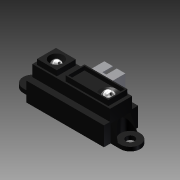
# Autodesk Inventor part: SharpIRsensor
Saved by Autodesk Inventor 2016 (Build 200138000, 138)
## iProperties
Created: 2012-10-14
Part Number: SharpIRsensor
Material: Ogólny
Document SubType Name: Modeling
Designer: ZSSD
Density: 1 g/cm^3
Appearance: Domyślna
Author: ZSSD
Autodesk Inventor part; units mm, degrees
sketch "Sketch1" plane through (0, 0, 0) normal (0, 0, 1) x (1, 0, 0)
  line L0 (0, 0) -> (29.5, 0)
  line L1 (29.5, 0) -> (29.5, 13)
  line L2 (29.5, 13) -> (0, 13)
  line L3 (0, 13) -> (0, 0)
  dimension "d0" = 29.5
  dimension "d1" = 13
  constraints: 8 end point, 2 parallel, 1 horizontal, 1 perpendicular
  measures "d0" distance of L2.end L1.end
  measures "d1" distance of L0.end L1.end
extrude "Extrusion1" add sketch "Sketch1" along normal blind 13.5
sketch "Sketch2" plane through (0, 0, 13.5) normal (0, 0, 1) x (1, 0, 0)
  line L0 (0, 0) -> (0, 13) projected
  line L1 (29.5, 13) -> (29.5, 0) projected
  line L2 (0, 6.5) -> (29.5, 6.5)
  line L3 (29.5, 6.5) -> (29.5, 10.7)
  line L4 (29.5, 10.7) -> (0, 10.7)
  line L5 (0, 10.7) -> (0, 6.5)
  line L6 (29.5, 10.7) -> (0, 10.7)
  line L7 (0, 10.7) -> (0, 2.3)
  line L8 (0, 2.3) -> (29.5, 2.3)
  line L9 (29.5, 2.3) -> (29.5, 10.7)
  dimension "d4" = 4.2
  dimension "d5" = 8.4
  constraints: 16 end point, 4 parallel, 2 horizontal, 2 perpendicular, 2 point on line, 1 midpoint
  measures "d4" distance of L3.end L2.end
  measures "d5" distance of L7.end L6.end
extrude "Extrusion2" add sketch "Sketch2" along normal blind 6.3
sketch "Sketch3" plane through (0, 0, 19.8) normal (0, 0, 1) x (1, 0, 0)
  line L0 (0, 2.3) -> (0, 10.7) projected
  line L1 (29.5, 2.3) -> (0, 2.3) projected
  line L2 (29.5, 10.7) -> (29.5, 2.3) projected
  line L3 (0, 10.7) -> (29.5, 10.7) projected
  line L4 (29.5, 6.5) -> (0, 6.5)
  line L5 (0, 6.5) -> (0, 10.1)
  line L6 (0, 10.1) -> (29.5, 10.1)
  line L7 (29.5, 10.1) -> (29.5, 6.5)
  line L8 (0, 10.1) -> (29.5, 10.1)
  line L9 (29.5, 10.1) -> (29.5, 2.9)
  line L10 (29.5, 2.9) -> (0, 2.9)
  line L11 (0, 2.9) -> (0, 10.1)
  line L12 (0, 10.7) -> (29.5, 10.7)
  line L13 (29.5, 10.7) -> (29.5, 10.1)
  line L14 (29.5, 10.1) -> (0, 10.1)
  line L15 (0, 10.1) -> (0, 10.7)
  point P0 (0, 0)
  dimension "d8" = 3.6
  dimension "d9" = 7.2
  constraints: 24 end point, 6 parallel, 3 horizontal, 3 perpendicular, 2 point on line, 1 midpoint
  measures "d8" distance of L4.end L5.end
  measures "d9" distance of L8.end L9.end
extrude "Extrusion3" cut sketch "Sketch3" against normal blind 2 contours L0 L10 L2 L1 | L0 L3 L2 L6
sketch "Sketch4" plane through (0, 0, 19.8) normal (0, 0, 1) x (1, 0, 0)
  line L0 (29.5, 10.1) -> (0, 10.1) projected
  line L1 (0, 2.9) -> (29.5, 2.9) projected
  line L2 (29.5, 2.9) -> (28.3, 2.9)
  line L3 (28.3, 2.9) -> (28.3, 10.1)
  line L4 (28.3, 10.1) -> (29.5, 10.1)
  line L5 (29.5, 10.1) -> (29.5, 2.9)
  line L6 (0, 10.1) -> (1.2, 10.1)
  line L7 (1.2, 10.1) -> (1.2, 2.9)
  line L8 (1.2, 2.9) -> (0, 2.9)
  line L9 (0, 2.9) -> (0, 10.1)
  point P0 (0, 0)
  dimension "d12" = 1.2
  dimension "d13" = 1.2
  constraints: 16 end point, 4 parallel, 2 horizontal, 2 perpendicular, 2 point on line
  measures "d12" distance of L3.end L4.end
  measures "d13" distance of L7.end L8.end
extrude "Extrusion4" cut sketch "Sketch4" against normal blind 2 contours L5 L1 L3 L0 | L7 L1 L9 L0
sketch "Sketch5" plane through (0, 0, 19.8) normal (0, 0, 1) x (1, 0, 0)
  line L0 (1.2, 2.9) -> (28.3, 2.9) projected
  line L1 (28.3, 10.1) -> (12, 10.1)
  line L2 (12, 10.1) -> (12, 2.9)
  line L3 (12, 2.9) -> (28.3, 2.9)
  line L4 (28.3, 2.9) -> (28.3, 10.1)
  line L5 (1.2, 10.1) -> (8.7, 10.1)
  line L6 (8.7, 10.1) -> (8.7, 2.9)
  line L7 (8.7, 2.9) -> (1.2, 2.9)
  line L8 (1.2, 2.9) -> (1.2, 10.1)
  line L9 (8.7, 10.1) -> (12, 10.1)
  line L10 (12, 10.1) -> (12, 2.9)
  line L11 (12, 2.9) -> (8.7, 2.9)
  line L12 (8.7, 2.9) -> (8.7, 10.1)
  point P0 (0, 0)
  dimension "d16" = 16.3
  dimension "d17" = 7.5
  constraints: 24 end point, 6 parallel, 3 horizontal, 3 perpendicular, 2 point on line
  measures "d16" distance of L3.end L2.end
  measures "d17" distance of L6.end L7.end
extrude "Extrusion5" cut sketch "Sketch5" against normal up to surface (2 mm away) contours L6 L9 L2 L0
sketch "Sketch6" plane through (0, 0, 0) normal (0, 0, -1) x (-1, 0, 0)
  line L0 (0, 0) -> (-29.5, 0) projected
  line L1 (0, 13) -> (0, 0) projected
  line L2 (-29.5, 13) -> (0, 13) projected
  line L3 (-29.5, 0) -> (-29.5, 13) projected
extrude "Extrusion6" cut sketch "Sketch6" against normal blind 6.3
sketch "Sketch7" plane through (0, 0, 6.3) normal (0, 0, -1) x (-1, 0, 0)
  line L0 (-29.5, 0) -> (-29.5, 13) projected
  line L1 (0, 0) -> (-29.5, 0) projected
  line L2 (-29.5, 6.2731) -> (-33.25, 6.2731)
  circle A0 centre (-33.25, 6.2731) radius 3.75
  circle A1 centre (-33.25, 6.2731) radius 1.6
  line L3 (-33.25, 10.0231) -> (-29.5, 10.0231)
  line L4 (-33.25, 2.5231) -> (-29.5, 2.5231)
  dimension "d22" = 3.75
  dimension "d23" = 3.2
  constraints: 6 end point, 3 point on circle, 3 point on line, 2 centre point, 2 coincident, 2 perpendicular, 2 tangent, 1 parallel
  measures "d22" distance of L2.start L2.end
  measures "d23" diameter of A1
extrude "Extrusion7" add sketch "Sketch7" against normal blind 1.5
sketch "Sketch8" plane through (0, 0, 7.8) normal (0, 0, 1) x (1, 0, 0)
  circle A0 centre (33.25, 6.2731) radius 1.6 projected
  line L0 (29.5, 10.0231) -> (33.25, 10.0231) projected
  line L1 (29.5, 2.5231) -> (29.5, 10.0231) projected
  line L2 (33.25, 2.5231) -> (29.5, 2.5231) projected
  arc A1 (33.25, 2.5231) -> (33.25, 10.0231) centre (33.25, 6.2731) ccw projected
  line L3 (29.5, 6.2731) -> (37, 6.2731)
  line L4 (33.25, 6.2731) -> (29.5, 6.2731)
  line L5 (29.5, 6.2731) -> (32.1, 6.2731)
  line L6 (32.1, 2.5231) -> (32.1, 10.0231)
  point P0 (0, 0)
  dimension "d26" = 2.6
  constraints: 8 end point, 3 point on line, 1 collinear, 1 midpoint, 1 perpendicular, 1 point on circle
  measures "d26" distance of L3.start L5.end
sketch "Sketch9" plane through (29.5, 10.7, 13.5) normal (1, 0, 0) x (0, 0, -1)
  line L0 (7.2, -8.1769) -> (5.7, -8.1769) projected
  line L1 (5.7, -8.1769) -> (5.7, -0.6769) projected
  line L2 (5.7, -0.6769) -> (7.2, -0.6769) projected
  line L3 (7.2, -0.6769) -> (7.2, 2.3) projected
  line L4 (7.2, 2.3) -> (0, 2.3) projected
  line L5 (0, 2.3) -> (0, 0) projected
  line L6 (0, 0) -> (-4.3, 0) projected
  line L7 (-4.3, 0) -> (-4.3, -8.4) projected
  line L8 (0, -8.4) -> (-4.3, -8.4) projected
  line L9 (0, -8.4) -> (0, -10.7) projected
  line L10 (7.2, -10.7) -> (0, -10.7) projected
  line L11 (7.2, -10.7) -> (7.2, -8.1769) projected
  line L12 (5.7, -8.1769) -> (0.7, -8.1769)
  line L13 (0.7, -8.1769) -> (0.7, -1.0276)
  line L14 (0.7, -1.0276) -> (5.7, -1.0276)
  line L15 (5.7, -1.0276) -> (5.7, -8.1769)
  point P0 (13.5, -10.7)
  dimension "d27" = 5
  constraints: 8 end point, 2 parallel, 1 horizontal, 1 perpendicular
  measures "d27" distance of L13.end L14.end
ref_plane "Work Plane1" through (31.375, 2.5231, 7.8) normal (0, -1, 0) x (1, 0, 0)
sketch "Sketch10" plane through (31.375, 2.5231, 7.8) normal (0, -1, 0) x (1, 0, 0)
  line L0 (-1.875, 0) -> (-1.875, 5) projected
  line L1 (1.875, 0) -> (-1.875, 0) projected
  line L2 (-1.875, 5) -> (0.725, 0)
  point P0 (-31.375, -7.8)
  constraints: 2 end point
extrude "Extrusion8" add sketch "Sketch10" against normal up to surface (7.5 mm away)
sketch "Sketch11" plane through (0, 0, 7.8) normal (0, 0, 1) x (1, 0, 0)
  arc A0 (33.25, 2.5231) -> (33.25, 10.0231) centre (33.25, 6.2731) ccw projected
  circle A1 centre (33.25, 6.2731) radius 3.75
  point P0 (0, 0)
  constraints: 1 centre point, 1 coincident, 1 concentric
extrude "Extrusion9" cut sketch "Sketch11" along normal through all
ref_plane "Work Plane2" through (14.75, 0, 13.5) normal (1, 0, 0) x (0, 0, -1)
mirror "Mirror1" about plane through (14.75, 0, 13.5) normal (1, 0, 0) of "Extrusion9", "Extrusion8", "Extrusion7"
sketch "Sketch12" plane through (0, 0, 19.8) normal (0, 0, 1) x (1, 0, 0)
  line L0 (1.2, 2.9) -> (8.7, 2.9) projected
  line L1 (4.95, 2.9) -> (4.95, 3.9)
  circle A0 centre (4.95, 6.5) radius 2.6
  point P0 (0, 0)
  dimension "d32" = 1
  constraints: 2 end point, 1 midpoint, 1 perpendicular, 1 vertical alignment, 2 other
  measures "d32" distance of L1.start L1.end
sketch "Sketch13" plane through (0, 0, 17.8) normal (0, 0, 1) x (1, 0, 0)
  circle A0 centre (4.95, 6.5) radius 1.75
  point P0 (0, 0)
  dimension "d33" = 3.5
  constraints: 1 centre point
  measures "d33" diameter of A0
loft "Loft1" cut profiles "Sketch13", "Sketch12"
sketch "Sketch14" plane through (4.95, 6.5, 17.8) normal (0, 0, 1) x (1, 0, 0)
  circle A0 centre (0, 0) radius 1.75 projected
  line L0 (-1.75, 0) -> (1.75, 0)
  point P0 (-4.95, -6.5)
  constraints: 2 end point, 2 point on circle, 1 horizontal
ref_plane "Work Plane3" through (0, 6.5, 13.5) normal (0, -1, 0) x (1, 0, 0)
sketch "Sketch15" plane through (0, 6.5, 13.5) normal (0, -1, 0) x (1, 0, 0)
  line L0 (3.2, 4.3) -> (6.7, 4.3) projected
  line L1 (3.2, 4.3) -> (6.7, 4.3)
  circle A0 centre (4.95, 4.3) radius 1.7743
  line L2 (6.7, 4.3) -> (3.1757, 4.3)
  arc A1 (6.7, 4.3) -> (3.1757, 4.3) centre (4.9379, 4.3121) ccw
  point P0 (0, -13.5)
  constraints: 4 end point, 2 point on circle, 1 centre point, 1 collinear, 1 horizontal alignment, 1 midpoint, 2 other
revolve "Revolution1" add sketch "Sketch15" angle 90 about axis through (3.2, 6.5, 17.8) along (1, 0, 0) picked at (5.5194, 4.4315) contours L2 A0 A1 L0 | A1 A0
sketch "Sketch16" plane through (3.2, 6.5, 17.8) normal (0, 1, 0) x (1, 0, 0)
  line L0 (-0.0238, -0.0559) -> (0, 0) projected
  arc A0 (-0.0238, -0.0559) -> (3.5, 0) centre (1.7379, -0.0121) ccw projected
  line L1 (0, 0) -> (3.5, 0) projected
  point P0 (-3.2, 17.8)
revolve "Revolution2" add sketch "Sketch16" angle 90 about axis through (3.2, 6.5, 17.8) along (-1, 0, 0)
sketch "Sketch17" plane through (0, 0, 19.8) normal (0, 0, 1) x (1, 0, 0)
  line L0 (12, 10.1) -> (12, 2.9) projected
  line L1 (12, 2.9) -> (28.3, 2.9) projected
  line L2 (28.3, 2.9) -> (28.3, 10.1) projected
  line L3 (28.3, 10.1) -> (12, 10.1) projected
  line L4 (13.3298, 10.1) -> (13.3298, 9.6)
  line L5 (12, 6.5) -> (12.5, 6.5)
  line L6 (25.802, 2.9) -> (25.802, 3.4)
  line L7 (28.3, 5.0475) -> (27.8, 5.0475)
  line L8 (12.5, 9.6) -> (27.8, 9.6)
  line L9 (27.8, 9.6) -> (27.8, 3.4)
  line L10 (27.8, 3.4) -> (12.5, 3.4)
  line L11 (12.5, 3.4) -> (12.5, 9.6)
  point P0 (0, 0)
  dimension "d40" = 0.5
  dimension "d41" = 0.5
  dimension "d42" = 0.5
  dimension "d43" = 0.5
  constraints: 16 end point, 5 perpendicular, 3 point on line, 2 parallel, 1 horizontal, 1 midpoint
  measures "d40" distance of L4.start L4.end
  measures "d41" distance of L5.start L5.end
  measures "d42" distance of L6.start L6.end
  measures "d43" distance of L7.start L7.end
extrude "Extrusion10" cut sketch "Sketch17" against normal blind 1.5 contours L11 L8 L9 L10
sketch "Sketch18" plane through (0, 0, 18.3) normal (0, 0, 1) x (1, 0, 0)
  line L0 (12.5, 3.4) -> (27.8, 3.4) projected
  line L1 (27.8, 9.6) -> (12.5, 9.6) projected
  line L2 (24.5676, 9.6) -> (24.5676, 3.4)
  circle A0 centre (24.6832, 6.5) radius 3.1
  line L3 (12.5, 9.6) -> (12.5, 3.4) projected
  line L4 (12.5, 3.4) -> (27.8, 3.4) projected
  line L5 (27.8, 3.4) -> (27.8, 9.6) projected
  line L6 (27.8, 9.6) -> (12.5, 9.6) projected
  line L7 (27.8, 9.6) -> (27.8, 3.4) projected
  line L8 (12.5, 9.6) -> (27.8, 9.6) projected
  line L9 (27.8, 9.6) -> (27.8, 3.4)
  point P0 (0, 0)
  dimension "d46" = 6.2
  constraints: 4 end point, 2 point on line, 1 centre point, 1 collinear, 1 perpendicular
  measures "d46" diameter of A0
sketch "Sketch19" plane through (0, 0, 17.8) normal (0, 0, 1) x (1, 0, 0)
  circle A0 centre (24.6832, 6.5) radius 2.1
  point P0 (0, 0)
  dimension "d47" = 4.2
  constraints: 1 centre point, 1 coincident
  measures "d47" diameter of A0
loft "Loft2" cut profiles "Sketch18", "Sketch19" contours A0 L2 | L2 A0 / all
sketch "Sketch20" plane through (24.6832, 6.5, 17.8) normal (0, 0, 1) x (1, 0, 0)
  circle A0 centre (0, 0) radius 2.1 projected
  point P0 (-24.6832, -6.5)
extrude "Extrusion11" cut sketch "Sketch20" against normal blind 0.5
sketch "Sketch21" plane through (0, 6.5, 13.5) normal (0, -1, 0) x (1, 0, 0)
  line L0 (26.7832, 3.8) -> (22.5832, 3.8) projected
  circle A0 centre (24.6832, 3.8) radius 2.1
  arc A1 (26.7832, 3.8) -> (22.5832, 3.8) centre (24.6832, 3.8) ccw
  line L1 (22.5832, 3.8) -> (26.7832, 3.8)
  point P0 (0, -13.5)
  constraints: 2 end point, 2 point on circle, 1 centre point, 1 collinear, 1 horizontal alignment, 1 midpoint, 3 other
revolve "Revolution3" add sketch "Sketch21" angle 360 about axis through (22.5832, 6.5, 17.3) along (1, 0, 0) picked at (24.9111, 4.622) contours L0 A0
sketch "Sketch22" plane through (0, 13, 13.5) normal (0, 1, 0) x (1, 0, 0)
  line L0 (29.5, 7.2) -> (0, 7.2) projected
  line L1 (29.5, 7.2) -> (29.5, 0) projected
  line L2 (14.75, 7.2) -> (14.75, 3.9)
  line L3 (14.75, 3.9) -> (19.8, 3.9)
  line L4 (19.8, 3.9) -> (19.8, 3.0162)
  line L5 (19.8, 3.0162) -> (14.75, 3.0162)
  line L6 (14.75, 3.0162) -> (14.75, 3.9)
  line L7 (19.8, 3.0162) -> (9.7, 3.0162)
  line L8 (9.7, 3.0162) -> (9.7, 3.9)
  line L9 (9.7, 3.9) -> (19.8, 3.9)
  line L10 (19.8, 3.9) -> (19.8, 3.0162)
  point P0 (0, 13.5)
  dimension "d55" = 3.3
  dimension "d56" = 5.05
  dimension "d57" = 10.1
  constraints: 18 end point, 5 parallel, 2 horizontal, 2 perpendicular, 1 midpoint
  measures "d55" distance of L2.start L2.end
  measures "d56" distance of L4.end L5.end
  measures "d57" distance of L8.end L9.end
extrude "Extrusion12" add sketch "Sketch22" along normal blind 5.9 contours L3 L4 L5 L6
sketch "Sketch23" plane through (14.75, 13, 10.4838) normal (0, 0, 1) x (1, 0, 0)
  line L0 (5.05, 0) -> (0, 0) projected
  line L1 (0, 5.9) -> (4, 5.9)
  line L2 (4, 5.9) -> (4, 0)
  line L3 (4, 0) -> (0, 0)
  line L4 (0, 0) -> (0, 5.9)
  point P0 (-14.75, -13)
  dimension "d60" = 4
  constraints: 8 end point, 2 parallel, 1 horizontal, 1 perpendicular, 1 point on line
  measures "d60" distance of L2.end L3.end
extrude "Extrusion13" add sketch "Sketch23" along normal blind 5.3
mirror "Mirror2" about plane through (14.75, 0, 13.5) normal (1, 0, 0) of "Extrusion13", "Extrusion12"
sketch "Sketch24" plane through (0, 18.9, 13.5) normal (0, 1, 0) x (1, 0, 0)
  line L0 (18.75, -2.2838) -> (10.75, -2.2838)
  line L1 (10.75, -2.2838) -> (10.75, 3.0162)
  line L2 (10.75, 3.0162) -> (18.75, 3.0162)
  line L3 (18.75, 3.0162) -> (18.75, -2.2838)
  line L4 (18.75, -2.2838) -> (19.4571, -2.2838) construction
  line L5 (10.75, 3.0162) -> (11.25, 2.5162)
  line L6 (18.75, -2.2838) -> (18.25, -1.7838)
  line L7 (18.25, -1.7838) -> (11.25, -1.7838)
  line L8 (11.25, -1.7838) -> (11.25, 2.5162)
  line L9 (11.25, 2.5162) -> (18.25, 2.5162)
  line L10 (18.25, 2.5162) -> (18.25, -1.7838)
  point P0 (0, 13.5)
  dimension "d65" = 0.5
  dimension "d66" = 0.5
  constraints: 22 end point, 5 parallel, 3 horizontal, 2 perpendicular
  measures "d65" horizontal distance of L1.end L5.end
  measures "d66" horizontal distance of L0.start L6.end
extrude "Extrusion14" cut sketch "Sketch24" against normal blind 4.5 contours L7 L8 L9 L10
sketch "Sketch25" plane through (18.75, 13, 10.4838) normal (1, 0, 0) x (0, 0, -1)
  line L0 (-5.3, 5.9) -> (-5.3, 0) projected
  line L1 (-3.0162, 0) -> (-5.3, 0) projected
  line L2 (0, 0) -> (-3.0162, 0) projected
  line L3 (0, 5.9) -> (0, 0) projected
  line L4 (0, 5.9) -> (-5.3, 5.9) projected
  line L5 (0, 0) -> (-5.3, 0)
  line L6 (0, 0) -> (-2.65, 0)
  line L7 (-2.65, 0) -> (-2.65, -2)
  line L8 (-2.65, -2) -> (-3.35, -2)
  line L9 (-3.0162, 0) -> (-5.3, 0)
  line L10 (-3.35, -2) -> (-4.1581, 0)
  point P0 (10.4838, -13)
  dimension "d69" = 2
  dimension "d70" = 0.7
  constraints: 12 end point, 2 midpoint, 2 perpendicular, 1 collinear, 1 parallel
  measures "d69" distance of L6.end L7.end
  measures "d70" distance of L7.end L8.end
extrude "Extrusion15" add sketch "Sketch25" against normal blind 0.5 contours L1 L2 L7 L8 L10
mirror "Mirror3" about plane through (14.75, 0, 13.5) normal (1, 0, 0) of "Extrusion15"
sketch "Sketch26" plane through (14.75, 13, 15.7838) normal (0, 0, 1) x (1, 0, 0)
  line L0 (-4, 5.9) -> (4, 5.9) projected
  line L1 (0, 5.9) -> (-0.75, 5.9)
  line L2 (-0.75, 5.9) -> (-0.75, 1.9)
  line L3 (-0.75, 1.9) -> (0, 1.9)
  line L4 (0, 1.9) -> (0, 5.9)
  line L5 (-0.75, 5.9) -> (0.75, 5.9)
  line L6 (0.75, 5.9) -> (0.75, 1.9)
  line L7 (0.75, 1.9) -> (-0.75, 1.9)
  line L8 (-0.75, 1.9) -> (-0.75, 5.9)
  point P0 (-14.75, -13)
  dimension "d73" = 0.75
  dimension "d74" = 4
  dimension "d75" = 1.5
  constraints: 16 end point, 4 parallel, 2 horizontal, 2 perpendicular, 1 midpoint
  measures "d73" distance of L3.end L2.end
  measures "d74" distance of L2.end L1.end
  measures "d75" distance of L6.end L7.end
extrude "Extrusion16" cut sketch "Sketch26" against normal blind 0.5
sketch "Sketch27" plane through (0, 0, 6.3) normal (0, 0, -1) x (-1, 0, 0)
  line L0 (-29.5, 13) -> (0, 13) projected
  line L1 (-29.5, 13) -> (-29, 12.5)
  line L2 (0, 0) -> (-0.5, 0.5)
  line L3 (-29, 12.5) -> (-0.5, 12.5)
  line L4 (-0.5, 12.5) -> (-0.5, 0.5)
  line L5 (-0.5, 0.5) -> (-29, 0.5)
  line L6 (-29, 0.5) -> (-29, 12.5)
  dimension "d78" = 45
  dimension "d79" = 0.5
  dimension "d80" = 0.5
  constraints: 12 end point, 3 parallel, 1 horizontal, 1 perpendicular
  measures "d78" angle of L0 L1
  measures "d79" horizontal distance of L0.start L1.end
  measures "d80" horizontal distance of L2.start L2.end
extrude "Extrusion17" cut sketch "Sketch27" against normal blind 3.3
body "Solid1"
